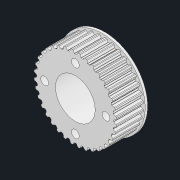
# Autodesk Inventor part: s3m-pulley1
Saved by Autodesk Inventor 2021 (Build 250183000, 183)
## iProperties
Created: 2021-07-14
Part Number: s3m-pulley1
Material: ABS プラスチック
Document SubType Name: Modeling
Designer: yuta0
Density: 1.06 g/cm^3
Appearance: 滑らか - 白
購入先: 印刷
在庫数: 0.0
Author: yuta0
Autodesk Inventor part; units mm, degrees
ref_plane "YZ Plane" through (0, 0, 0) normal (1, 0, 0) x (0, 1, 0)
ref_plane "XZ Plane" through (0, 0, 0) normal (0, 1, 0) x (-1, 0, 0)
ref_plane "XY Plane" through (0, 0, 0) normal (0, 0, 1) x (1, 0, 0)
sketch "スケッチ1" plane through (0, 0, 0) normal (0, 0, 1) x (1, 0, 0)
  circle A0 centre (0, 0) radius 17.1887 construction
  circle A1 centre (0, 0) radius 16.8077
  circle A2 centre (0, 0) radius 15.6977
  line L0 (-0.975, 17.1611) -> (0.975, 17.1611) construction
  line L1 (-24.0642, 0) -> (24.0642, 0) projected
  circle A3 centre (0.975, 17.1611) radius 1.975
  circle A4 centre (-0.975, 17.1611) radius 1.975
  point P0 (0, 16.8077)
  point P1 (0.3471, 15.6939)
  point P2 (0.9629, 16.7801)
  point P3 (-0.9629, 16.7801)
  point P4 (-0.3471, 15.6939)
  point P5 (0, 16.8077)
  dimension "d1" = 34.3775
  dimension "d2" = 0.381
  dimension "d3" = 1.11
  dimension "d5" = 3.95
  dimension "d6" = 1.95
  dimension "d7" = 3.95
  constraints: 4 centre point, 4 coincident, 2 end point, 2 point on circle, 1 parallel, 1 vertical alignment, 3 other
  measures "d1" diameter of A0
  measures "d5" diameter of A3
  measures "d6" distance of L0.start L0.end
  measures "d7" diameter of A4
extrude "押し出し1" add sketch "スケッチ1" against normal blind 11 contours L1 A2 A3 A1 | A1 L1 A2 | A3 A2 A4 A1 | A1 A4 A2 L1 | L1 A2 A4 A3 | A2 L1 | A4 A2 A3 A1 | A3 A4 A2 | A1 A3 A2 A4 | A4 A3 A2 | A4 A2 A3
extrude "押し出し2" cut sketch "スケッチ1" against normal through all contours A4 A2 A3 A1 picked at (-0.0386, 16.4355)
fillet "フィレット1" radius 0.285 2 edges at (0.9629, 16.7801, -5.5) (-0.9629, 16.7801, -5.5)
fillet "フィレット2" radius 0.15 2 edges at (0.3471, 15.6939, -5.5) (-0.3471, 15.6939, -5.5)
pattern_circular "円形状パターン1" count 36 over 360 about axis through (0, 0, -10) along (0, 0, 1) of "押し出し2", "フィレット1", "フィレット2"
sketch "スケッチ9" plane through (0, 0, -11) normal (0, 0, -1) x (-1, 0, 0)
  circle A0 centre (0, 0) radius 17.5 projected
extrude "押し出し8" add sketch "スケッチ9" along normal blind 1
sketch "スケッチ2" plane through (0, 0, -12) normal (0, 0, -1) x (1, 0, 0)
  circle A0 centre (0, 0) radius 12.5
  point P0 (0, 12.5)
  point P1 (-12.5, 0)
  point P2 (0, -12.5)
  point P3 (12.5, 0)
  dimension "d17" = 25
  dimension "d20" = 360
  constraints: 1 coincident, 1 vertical alignment, 7 other
hole "穴1" at (12.5, 0, -12) at (0, 12.5, -12) at (-12.5, 0, -12) at (0, -12.5, -12) direction (0, 0, 1) diameter 3.2 end through all clearance for "Socket Head Cap Screw" size "M3" standard "Ansi Metric M Profile"
sketch "スケッチ6" plane through (0, 0, -12) normal (0, 0, 1) x (1, 0, 0)
  circle A0 centre (0, 0) radius 8.1
  dimension "d48" = 16.2
  constraints: 1 centre point, 1 coincident
  measures "d48" diameter of A0
extrude "押し出し5" cut sketch "スケッチ6" along normal through all
equation "\"d7\" = d5"
